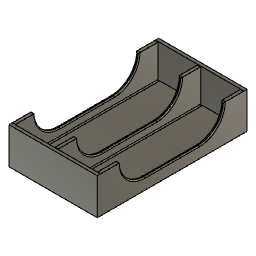
battery-case (Autodesk Fusion 360 design; units mm, degrees)
Autodesk Fusion 360 part; units mm, degrees
sketch "Sketch1" plane through (0, 0, 0) normal (0, 0, 1) x (1, 0, 0)
  line L0 (25, 25) -> (67.5, 25)
  line L1 (67.5, 25) -> (67.5, 97)
  line L2 (67.5, 97) -> (25, 97)
  line L3 (25, 97) -> (25, 25)
  dimension "d1" = 42.5
  dimension "d2" = 72
  constraint horizontal L0
  constraint vertical L1
  constraint horizontal L2
  constraint vertical L3
  measures "d1" distance of L0.start L0.end
  measures "d2" distance of L0.start L2.end
extrude "Extrude1" add sketch "Sketch1" along normal blind 17.5
sketch "Sketch2" plane through (0, 0, 17.5) normal (0, 0, 1) x (-1, 0, 0)
  line L0 (-25, -97) -> (-25, -25)
  line L1 (-25, -25) -> (-67.5, -25)
  line L2 (-67.5, -25) -> (-67.5, -97)
  line L3 (-67.5, -97) -> (-25, -97)
  line L4 (-25, -97) -> (-26.5, -97)
  line L5 (-26.5, -97) -> (-26.5, -95.5)
  line L6 (-26.5, -95.5) -> (-25, -95.5)
  line L7 (-25, -95.5) -> (-25, -97)
  line L8 (-67.5, -25) -> (-66, -25)
  line L9 (-66, -25) -> (-66, -26.5)
  line L10 (-66, -26.5) -> (-67.5, -26.5)
  line L11 (-67.5, -26.5) -> (-67.5, -25)
  line L12 (-47, -25) -> (-45.5, -25) construction
  line L13 (-45.5, -25) -> (-45.5, -26.5) construction
  line L14 (-45.5, -26.5) -> (-47, -26.5) construction
  line L15 (-47, -26.5) -> (-47, -25) construction
  line L16 (-26.5, -95.5) -> (-45.5, -95.5)
  line L17 (-45.5, -95.5) -> (-45.5, -26.5)
  line L18 (-45.5, -26.5) -> (-26.5, -26.5)
  line L19 (-26.5, -26.5) -> (-26.5, -95.5)
  line L20 (-45.5, -97) -> (-47, -97)
  line L21 (-47, -97) -> (-47, -95.5)
  line L22 (-47, -95.5) -> (-45.5, -95.5)
  line L23 (-45.5, -95.5) -> (-45.5, -97)
  line L24 (-47, -95.5) -> (-66, -95.5)
  line L25 (-66, -95.5) -> (-66, -26.5)
  line L26 (-66, -26.5) -> (-47, -26.5)
  line L27 (-47, -26.5) -> (-47, -95.5)
  point P0 (-47, -25)
  point P1 (-45.5, -97)
  dimension "d5" = 1.5
  dimension "d6" = 1.5
  dimension "d7" = 1.5
  dimension "d8" = 1.5
  dimension "d9" = 22
  dimension "d10" = 1.5
  dimension "d11" = 1.5
  dimension "d12" = 22
  dimension "d15" = 1.5
  dimension "d16" = 1.5
  constraint horizontal L4
  constraint vertical L5
  constraint horizontal L6
  constraint vertical L7
  constraint coincident L0.start L3.end
  constraint horizontal L8
  constraint vertical L9
  constraint horizontal L10
  constraint vertical L11
  constraint coincident L1.end L2.start
  constraint coincident L1 P0
  constraint coincident L3 P1
  constraint horizontal L12
  constraint vertical L13
  constraint horizontal L14
  constraint vertical L15
  constraint coincident P0 L12.start
  constraint horizontal L16
  constraint vertical L17
  constraint horizontal L18
  constraint vertical L19
  constraint horizontal L20
  constraint vertical L21
  constraint horizontal L22
  constraint vertical L23
  constraint coincident P1 L20.start
  constraint horizontal L24
  constraint vertical L25
  constraint horizontal L26
  constraint vertical L27
  measures "d5" distance of L0.start L4.end
  measures "d6" distance of L0.start L6.end
  measures "d7" distance of L1.end L8.end
  measures "d8" distance of L1.end L10.end
  measures "d9" distance of L0.end P0
  measures "d10" distance of P0 L12.end
  measures "d11" distance of P0 L14.end
  measures "d12" distance of L2.end P1
  measures "d15" distance of P1 L20.end
  measures "d16" distance of P1 L16.end
extrude "Extrude2" cut sketch "Sketch2" against normal blind 16 contours L16 L17 L18 L19 | L24 L25 L26 L27
sketch "Sketch3" plane through (25, 0, 0) normal (-1, 0, 0) x (0, -1, 0)
  line L0 (-97, 0) -> (-25, 0)
  line L1 (-25, 0) -> (-25, 17.5)
  line L2 (-25, 17.5) -> (-97, 17.5)
  line L3 (-97, 17.5) -> (-97, 0)
  line L4 (-61, 0) -> (-61, 17.5) construction
  line L5 (-74, 5.5) -> (-48, 5.5)
  arc A0 (-48, 5.5) -> (-48, 29.5) centre (-48, 17.5) ccw
  line L6 (-48, 29.5) -> (-74, 29.5)
  arc A1 (-74, 29.5) -> (-74, 5.5) centre (-74, 17.5) ccw
  line L7 (-86, 17.5) -> (-36, 17.5) construction
  point P0 (-36, 17.5)
  point P1 (-86, 17.5)
  dimension "d19" = 25
  dimension "d20" = 25
  dimension "d21" = 24
  constraint midpoint L0 L4.start
  constraint midpoint L2 L4.end
  constraint coincident L2 P0
  constraint coincident L2 P1
  constraint tangent L5 A0
  constraint tangent A0 L6
  constraint parallel L5 L6
  constraint tangent L6 A1
  constraint tangent L5 A1
  constraint midpoint A1 P1
  constraint midpoint A0 P0
  constraint coincident P0 L7.end
  constraint perpendicular L1 L7
  constraint coincident P1 L7.start
  measures "d19" distance of L4.end P1
  measures "d20" distance of L4.end P0
  measures "d21" diameter of A0
extrude "Extrude3" cut sketch "Sketch3" against normal blind 42.5 contours L2 L5 A0 A1
fillet "Fillet1" radius 0.5 24 edges at (25, 39.5147, 9.0147) (25, 61, 5.5) (25, 82.4853, 9.0147) (45.5, 39.5147, 9.0147) (45.5, 61, 5.5) (45.5, 82.4853, 9.0147) (66, 39.5147, 9.0147) (66, 61, 5.5) (66, 82.4853, 9.0147) (26.5, 82.4853, 9.0147) (26.5, 61, 5.5) (26.5, 39.5147, 9.0147) (47, 82.4853, 9.0147) (47, 61, 5.5) (47, 39.5147, 9.0147) (67.5, 82.4853, 9.0147) (67.5, 61, 5.5) (67.5, 39.5147, 9.0147) (66.75, 36, 17.5) (46.25, 36, 17.5) (25.75, 36, 17.5) (25.75, 86, 17.5) (46.25, 86, 17.5) (66.75, 86, 17.5)
sketch "Sketch4" plane through (0, 0, 17.5) normal (0, 0, 1) x (-1, 0, 0)
  arc A0 (-67.4999, -86.49) -> (-67.5, -86.5) centre (-67, -86.5) ccw
  line L0 (-67.5, -86.5) -> (-67.5, -97)
  line L1 (-67.5, -97) -> (-25, -97)
  line L2 (-25, -97) -> (-25, -86.5)
  arc A1 (-25, -86.5) -> (-25.0001, -86.49) centre (-25.5, -86.5) ccw
  line L3 (-25.0001, -86.49) -> (-26.4999, -86.49)
  arc A2 (-26.4999, -86.49) -> (-26.5, -86.5) centre (-26, -86.5) ccw
  line L4 (-26.5, -86.5) -> (-26.5, -95.5)
  line L5 (-26.5, -95.5) -> (-45.5, -95.5)
  line L6 (-45.5, -95.5) -> (-45.5, -86.5)
  arc A3 (-45.5, -86.5) -> (-45.5001, -86.49) centre (-46, -86.5) ccw
  line L7 (-45.5001, -86.49) -> (-46.9999, -86.49)
  arc A4 (-46.9999, -86.49) -> (-47, -86.5) centre (-46.5, -86.5) ccw
  line L8 (-47, -86.5) -> (-47, -95.5)
  line L9 (-47, -95.5) -> (-66, -95.5)
  line L10 (-66, -95.5) -> (-66, -86.5)
  arc A5 (-66, -86.5) -> (-66.0001, -86.49) centre (-66.5, -86.5) ccw
  line L11 (-66.0001, -86.49) -> (-67.4999, -86.49)
  line L12 (-26.5, -95.5) -> (-25.5, -95.5)
  line L13 (-25.5, -95.5) -> (-25.5, -95.2)
  line L14 (-25.5, -95.2) -> (-26.5, -95.2)
  line L15 (-26.5, -95.2) -> (-26.5, -95.5)
  line L16 (-66, -95.5) -> (-67, -95.5)
  line L17 (-67, -95.5) -> (-67, -95.2)
  line L18 (-67, -95.2) -> (-66, -95.2)
  line L19 (-66, -95.2) -> (-66, -95.5)
  line L20 (-45.5, -95.5) -> (-46.15, -95.5)
  line L21 (-46.15, -95.5) -> (-46.15, -95.2)
  line L22 (-46.15, -95.2) -> (-45.5, -95.2)
  line L23 (-45.5, -95.2) -> (-45.5, -95.5)
  line L24 (-47, -95.5) -> (-46.35, -95.5)
  line L25 (-46.35, -95.5) -> (-46.35, -95.2)
  line L26 (-46.35, -95.2) -> (-47, -95.2)
  line L27 (-47, -95.2) -> (-47, -95.5)
  dimension "d25" = 1
  dimension "d26" = 0.3
  dimension "d27" = 1
  dimension "d28" = 0.3
  dimension "d29" = 0.65
  dimension "d30" = 0.3
  dimension "d42" = 0.65
  dimension "d43" = 0.3
  constraint horizontal L12
  constraint vertical L13
  constraint horizontal L14
  constraint vertical L15
  constraint coincident L4.end L5.start
  constraint horizontal L16
  constraint vertical L17
  constraint horizontal L18
  constraint vertical L19
  constraint coincident L9.end L10.start
  constraint horizontal L20
  constraint vertical L21
  constraint horizontal L22
  constraint vertical L23
  constraint coincident L5.end L6.start
  constraint horizontal L24
  constraint vertical L25
  constraint horizontal L26
  constraint vertical L27
  constraint coincident L8.end L9.start
  measures "d25" distance of L4.end L12.end
  measures "d26" distance of L4.end L14.end
  measures "d27" distance of L9.end L16.end
  measures "d28" distance of L9.end L18.end
  measures "d29" distance of L5.end L20.end
  measures "d30" distance of L5.end L22.end
  measures "d42" distance of L8.end L24.end
  measures "d43" distance of L8.end L26.end
sketch "Sketch5" plane through (0, 0, 17.5) normal (0, 0, 1) x (-1, 0, 0)
  arc A0 (-67.5, -35.5) -> (-67.4999, -35.51) centre (-67, -35.5) ccw
  line L0 (-67.4999, -35.51) -> (-66.0001, -35.51)
  arc A1 (-66.0001, -35.51) -> (-66, -35.5) centre (-66.5, -35.5) ccw
  line L1 (-66, -35.5) -> (-66, -26.5)
  line L2 (-66, -26.5) -> (-47, -26.5)
  line L3 (-47, -26.5) -> (-47, -35.5)
  arc A2 (-47, -35.5) -> (-46.9999, -35.51) centre (-46.5, -35.5) ccw
  line L4 (-46.9999, -35.51) -> (-45.5001, -35.51)
  arc A3 (-45.5001, -35.51) -> (-45.5, -35.5) centre (-46, -35.5) ccw
  line L5 (-45.5, -35.5) -> (-45.5, -26.5)
  line L6 (-45.5, -26.5) -> (-26.5, -26.5)
  line L7 (-26.5, -26.5) -> (-26.5, -35.5)
  arc A4 (-26.5, -35.5) -> (-26.4999, -35.51) centre (-26, -35.5) ccw
  line L8 (-26.4999, -35.51) -> (-25.0001, -35.51)
  arc A5 (-25.0001, -35.51) -> (-25, -35.5) centre (-25.5, -35.5) ccw
  line L9 (-25, -35.5) -> (-25, -25)
  line L10 (-25, -25) -> (-67.5, -25)
  line L11 (-67.5, -25) -> (-67.5, -35.5)
  line L12 (-26.5, -26.5) -> (-25.5, -26.5)
  line L13 (-25.5, -26.5) -> (-25.5, -26.8)
  line L14 (-25.5, -26.8) -> (-26.5, -26.8)
  line L15 (-26.5, -26.8) -> (-26.5, -26.5)
  line L16 (-45.5, -26.5) -> (-46.15, -26.5)
  line L17 (-46.15, -26.5) -> (-46.15, -26.8)
  line L18 (-46.15, -26.8) -> (-45.5, -26.8)
  line L19 (-45.5, -26.8) -> (-45.5, -26.5)
  line L20 (-47, -26.5) -> (-46.35, -26.5)
  line L21 (-46.35, -26.5) -> (-46.35, -26.8)
  line L22 (-46.35, -26.8) -> (-47, -26.8)
  line L23 (-47, -26.8) -> (-47, -26.5)
  line L24 (-66, -26.5) -> (-66.7, -26.5)
  line L25 (-66.7, -26.5) -> (-66.7, -26.8)
  line L26 (-66.7, -26.8) -> (-66, -26.8)
  line L27 (-66, -26.8) -> (-66, -26.5)
  dimension "d31" = 1
  dimension "d32" = 0.3
  dimension "d33" = 0.65
  dimension "d34" = 0.3
  dimension "d35" = 0.65
  dimension "d36" = 0.3
  dimension "d37" = 0.7
  dimension "d38" = 0.3
  constraint horizontal L12
  constraint vertical L13
  constraint horizontal L14
  constraint vertical L15
  constraint coincident L6.end L7.start
  constraint horizontal L16
  constraint vertical L17
  constraint horizontal L18
  constraint vertical L19
  constraint coincident L5.end L6.start
  constraint horizontal L20
  constraint vertical L21
  constraint horizontal L22
  constraint vertical L23
  constraint coincident L2.end L3.start
  constraint horizontal L24
  constraint vertical L25
  constraint horizontal L26
  constraint vertical L27
  constraint coincident L1.end L2.start
  measures "d31" distance of L6.end L12.end
  measures "d32" distance of L6.end L14.end
  measures "d33" distance of L5.end L16.end
  measures "d34" distance of L5.end L18.end
  measures "d35" distance of L2.end L20.end
  measures "d36" distance of L2.end L22.end
  measures "d37" distance of L1.end L24.end
  measures "d38" distance of L1.end L26.end
extrude "Extrude4" cut sketch "Sketch4" sketch "Sketch5" against normal blind 16 contours L10 L16 L17 L18 L19 | L8 L24 L25 L26 L27 | L4 L12 L13 L14 L15 | L6 L20 L21 L22 L23 of sketch 2 contours L1 L24 L25 L26 L27 | L3 L20 L21 L22 L23 | L7 L12 L13 L14 L15 | L5 L16 L17 L18 L19
fillet "Fillet2" radius 0.5 4 edges at (26.5, 61, 1.5) (45.5, 61, 1.5) (47, 61, 1.5) (66, 61, 1.5)
